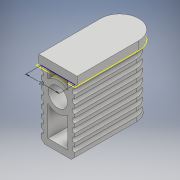
# Autodesk Inventor part: Kontorstol_hjulholder
Saved by Autodesk Inventor 2018 (Build 220112000, 112)
## iProperties
Created: 2019-02-04
Part Number: Kontorstol_hjulholder
Material: Generic
Document SubType Name: Modeling
Designer: JARVIS
Density: 1 g/cm^3
Appearance: Default
Author: JARVIS
Autodesk Inventor part; units mm, degrees
ref_plane "YZ Plane" through (0, 0, 0) normal (1, 0, 0) x (0, 1, 0)
ref_plane "XZ Plane" through (0, 0, 0) normal (0, 1, 0) x (-1, 0, 0)
ref_plane "XY Plane" through (0, 0, 0) normal (0, 0, 1) x (1, 0, 0)
sketch "Sketch1" plane through (0, 0, 0) normal (0, 0, 1) x (1, 0, 0)
  line L0 (-11.5, 0) -> (11.5, 0)
  line L1 (11.5, 0) -> (11.5, 38.5)
  arc A0 (11.5, 38.5) -> (-11.5, 38.5) centre (0, 38.5) ccw
  line L2 (-11.5, 38.5) -> (-11.5, 0)
  point P0 (0, 0)
  point P1 (0, 0)
  dimension "d0" = 38.5
  dimension "d1" = 11.5
  constraints: 6 end point, 2 coincident, 2 point on circle, 1 centre point, 1 horizontal, 1 midpoint, 1 parallel, 1 perpendicular, 1 tangent, 1 vertical alignment
  measures "d0" distance of A0.centre point (0, 0)
  measures "d1" radius of A0
extrude "Extrusion1" add sketch "Sketch1" along normal blind 5
sketch "Sketch2" plane through (0, 0, 0) normal (0, 0, -1) x (-1, 0, 0)
  line L0 (11.5, 0) -> (-11.5, 0) projected
  line L1 (11.5, 38.5) -> (11.5, 0) projected
  arc A0 (11.5, 38.5) -> (-11.5, 38.5) centre (0, 38.5) ccw projected
  line L2 (-11.5, 0) -> (-11.5, 38.5) projected
  arc A1 (10, 38.5) -> (-10, 38.5) centre (0, 38.5) ccw
  line L3 (10, 38.5) -> (10, 1.5)
  line L4 (10, 1.5) -> (-10, 1.5)
  line L5 (-10, 1.5) -> (-10, 38.5)
  point P0 (0, 0)
  dimension "d4" = 20
  constraints: 6 end point, 2 point on circle, 1 centre point, 3 other
  measures "d4" distance between parallel lines of L3 L5
extrude "Extrusion2" add sketch "Sketch2" along normal blind 40 contours L3 L4 L5 A1
sketch "Sketch3" plane through (-10, 1.5, 0) normal (0, -1, 0) x (1, 0, 0)
  line L0 (0, 0) -> (20, 0) projected
  line L1 (0, 0) -> (0, -40) projected
  line L2 (20, -40) -> (0, -40) projected
  line L3 (20, 0) -> (20, -40) projected
  circle A0 centre (10, -11.5) radius 5.75
  arc A1 (5.8824, -3.7794) -> (4, -5.1311) centre (10, -11.5) ccw
  line L4 (-1.5, 0) -> (21.5, 0) projected
  arc A2 (14.1176, -3.7794) -> (5.8824, -3.7794) centre (10, -11.5) ccw
  arc A3 (3.8235, -5.3021) -> (4, -17.8689) centre (10, -11.5) ccw
  line L5 (4, 0) -> (16, 0)
  line L6 (16, 0) -> (16, -17.8689)
  line L7 (16, -36) -> (4, -36)
  line L8 (4, -36) -> (4, -17.8689)
  arc A4 (4, -5.1311) -> (3.8235, -5.3021) centre (10, -11.5) ccw
  arc A5 (16, -5.1311) -> (14.1176, -3.7794) centre (10, -11.5) ccw
  line L9 (16, -17.8689) -> (16, -36)
  arc A6 (4, -17.8689) -> (16, -17.8689) centre (10, -11.5) ccw
  line L10 (4, 0) -> (16, 0)
  line L11 (4, -17.8689) -> (4, 0)
  arc A7 (16, -17.8689) -> (16, -5.1311) centre (10, -11.5) ccw
  point P0 (10, 0)
  point P1 (10, 0)
  point P2 (16.1765, -17.6979)
  point P3 (3.8235, -17.6979)
  dimension "d8" = 11.5
  dimension "d9" = 3
  dimension "d10" = 11.5
  dimension "d31" = 4
  dimension "d32" = 4
  dimension "d33" = 4
  constraints: 23 point on circle, 14 end point, 8 centre point, 5 parallel, 4 point on line, 2 perpendicular, 1 coincident, 1 collinear, 1 horizontal, 1 midpoint, 1 vertical alignment
  measures "d8" diameter of A0
  measures "d9" radial gap between concentric circles of A1 A0
  measures "d10" distance of point (10, 0) A0.centre
  measures "d31" distance between parallel lines of L2 L7
  measures "d32" distance between parallel lines of L3 L6
  measures "d33" distance between parallel lines of L8 L1
extrude "Extrusion3" cut sketch "Sketch3" against normal blind 40 contours L0 L6 A5 A2 A1 L11 | A6 L9 L7 L8 | A0
sketch "Sketch4" plane through (-10, 1.5, 0) normal (0, -1, 0) x (1, 0, 0)
  line L0 (20, 0) -> (20, -40) projected
  line L1 (0, 0) -> (0, -40) projected
  line L2 (0, 0) -> (4, 0) projected
  line L3 (0, 0) -> (0, -40) projected
  line L4 (20, -40) -> (0, -40) projected
  line L5 (20, 0) -> (20, -40) projected
  line L6 (20, -40) -> (0, -40) projected
  line L7 (18.5, 0) -> (18.5, -38.5)
  line L8 (18.5, -38.5) -> (1.5, -38.5)
  line L9 (1.5, -38.5) -> (1.5, 0)
  circle A0 centre (20, -33.9327) radius 1.5
  line L10 (20, 0) -> (20, -40) projected
  circle A1 centre (20, -28.9327) radius 1.5
  circle A2 centre (20, -23.9327) radius 1.5
  circle A3 centre (20, -18.9327) radius 1.5
  circle A4 centre (20, -13.9327) radius 1.5
  circle A5 centre (20, -8.9327) radius 1.5
  circle A6 centre (20, -3.9327) radius 1.5
  line L11 (16, 0) -> (20, 0) projected
  line L12 (16, 0) -> (16, -5.1311) projected
  arc A7 (16, -5.1311) -> (4, -5.1311) centre (10, -11.5) ccw projected
  line L13 (4, -5.1311) -> (4, 0) projected
  point P0 (10, 0)
  dimension "d13" = 17
  dimension "d14" = 5
  dimension "d15" = 5
  dimension "d16" = 5
  dimension "d17" = 5
  dimension "d18" = 5
  dimension "d19" = 5
  constraints: 7 centre point, 7 point on line, 6 end point, 6 tangent, 2 other
  measures "d13" distance between parallel lines of L9 L7
  measures "d14" distance of A5.centre A6.centre
  measures "d15" distance of A4.centre A5.centre
  measures "d16" distance of A3.centre A4.centre
  measures "d17" distance of A2.centre A3.centre
  measures "d18" distance of A1.centre A2.centre
  measures "d19" distance of A0.centre A1.centre
extrude "Extrusion4" cut sketch "Sketch4" against normal through all contours A6 L0 | L0 A6 | A5 L0 | L0 A5 | A4 L0 | A4 L0 | A3 L0 | A2 L0 | A3 L0 | A1 L0 | A2 L0 | A0 L0 | A1 L0 | A0 L0
mirror "Mirror1" about plane through (0, 0, 0) normal (1, 0, 0) of "Extrusion4"
chamfer "Chamfer1" distance 2 angle 45 3 edges at (10, 20, -40) (0, 48.5, -40) (-10, 20, -40)
chamfer "Chamfer2" distance 4 angle 45 1 edges at (-5.75, 41.5, -11.5)
sketch "Sketch5" plane through (0, 0, 0) normal (0, 0, -1) x (-1, 0, 0)
  line L0 (11.5, 0) -> (-11.5, 0) projected
  line L1 (-11.5, 0) -> (-11.5, 38.5) projected
  line L2 (11.5, 0) -> (-11.5, 0)
  line L3 (-11.5, 0) -> (-11.5, 1.5)
  line L4 (-11.5, 1.5) -> (11.5, 1.5)
  line L5 (11.5, 1.5) -> (11.5, 0)
  line L6 (-8, 1.5) -> (8, 1.5) projected
  point P0 (0, 0)
  point P1 (0, 1.5)
  constraints: 8 end point, 2 parallel, 1 horizontal, 1 horizontal alignment, 1 midpoint, 1 perpendicular, 1 point on line
extrude "Extrusion5" cut sketch "Sketch5" against normal blind 40
equation "\"d15\" = d14"
equation "\"d16\" = d14"
equation "\"d17\" = d14"
equation "\"d18\" = d14"
equation "\"d19\" = d14"
body "Solid1"
